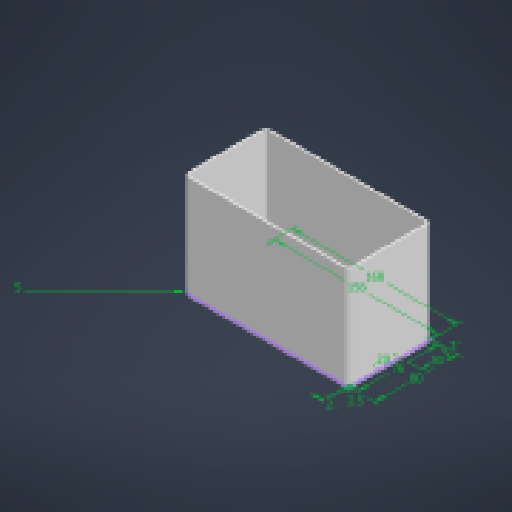
# Autodesk Inventor part: Base
Saved by Autodesk Inventor 2026.1 (Build 301233020, 233B)
## iProperties
Created: 2025-10-20
Part Number: Base
Material: Generic
Document SubType Name: Modeling
Designer: Nathan
Density: 1 g/cm^3
Appearance: Default
Author: Nathan
Autodesk Inventor part; units mm, degrees
ref_plane "YZ Plane" through (0, 0, 0) normal (1, 0, 0) x (0, 1, 0)
ref_plane "XZ Plane" through (0, 0, 0) normal (0, 1, 0) x (-1, 0, 0)
ref_plane "XY Plane" through (0, 0, 0) normal (0, 0, 1) x (1, 0, 0)
sketch "BaseBottom" plane through (0, 0, 0) normal (0, 1, 0) x (-1, 0, 0)
  line L0 (108.8151, 0.0203) -> (-41.1849, 0.0203)
  line L1 (-46.1849, -4.9797) -> (-46.1849, -74.9797)
  line L2 (-41.1849, -79.9797) -> (108.8151, -79.9797)
  line L3 (113.8151, -74.9797) -> (113.8151, -4.9797)
  arc A0 (113.8151, -4.9797) -> (108.8151, 0.0203) centre (108.8151, -4.9797) ccw
  arc A1 (108.8151, -79.9797) -> (113.8151, -74.9797) centre (108.8151, -74.9797) ccw
  arc A2 (-46.1849, -74.9797) -> (-41.1849, -79.9797) centre (-41.1849, -74.9797) ccw
  arc A3 (-41.1849, 0.0203) -> (-46.1849, -4.9797) centre (-41.1849, -4.9797) ccw
  line L4 (109.3151, -1.9797) -> (-41.6849, -1.9797)
  line L5 (-44.1849, -4.4797) -> (-44.1849, -75.4797)
  line L6 (-41.6849, -77.9797) -> (109.3151, -77.9797)
  line L7 (111.8151, -75.4797) -> (111.8151, -4.4797)
  arc A4 (-41.6849, -1.9797) -> (-44.1849, -4.4797) centre (-41.6849, -4.4797) ccw
  arc A5 (-44.1849, -75.4797) -> (-41.6849, -77.9797) centre (-41.6849, -75.4797) ccw
  arc A6 (109.3151, -77.9797) -> (111.8151, -75.4797) centre (109.3151, -75.4797) ccw
  arc A7 (111.8151, -4.4797) -> (109.3151, -1.9797) centre (109.3151, -4.4797) ccw
  line L8 (-46.1849, -29.9797) -> (-44.1849, -29.9797)
  line L9 (-44.1849, -29.9797) -> (-44.1849, -49.9797)
  line L10 (-44.1849, -49.9797) -> (-46.1849, -49.9797)
  line L11 (-46.1849, -49.9797) -> (-46.1849, -29.9797)
  point P0 (-46.1849, -79.9797)
  point P1 (-46.1849, 0.0203)
  point P2 (113.8151, -79.9797)
  point P3 (-44.1849, -77.9797)
  point P4 (-44.1849, -1.9797)
  point P5 (111.8151, -77.9797)
  point P6 (-45.1849, -49.9797)
  dimension "d2" = 160
  dimension "d3" = 80
  dimension "d4" = 5
  dimension "d6" = 156
  dimension "d7" = 76
  dimension "d8" = 2
  dimension "d9" = 2
  dimension "d10" = 2.5
  dimension "d11" = 20
  dimension "d12" = 30
  constraints: 24 end point, 16 point on circle, 16 tangent, 14 point on line, 8 centre point, 6 equal radius, 6 parallel, 3 horizontal, 3 perpendicular, 1 midpoint
  measures "d2" distance of point (113.815, -79.98) point (-46.185, -79.98)
  measures "d3" distance of point (-46.185, -79.98) point (-46.185, 0.02)
  measures "d4" radius of A0
  measures "d6" distance of point (111.815, -77.98) point (-44.185, -77.98)
  measures "d7" distance of point (-44.185, -77.98) point (-44.185, -1.98)
  measures "d8" distance between parallel lines of L2 L6
  measures "d9" distance between parallel lines of L1 L5
  measures "d10" radius of A4
  measures "d11" distance of L8.end L9.end
  measures "d12" distance from line of L2 point (-45.185, -49.98)
extrude "BaseFloor" add sketch "BaseBottom" against normal blind 2
extrude "BaseFill" add sketch "BaseBottom" along normal blind 98
extrude "BaseHollow" cut sketch "BaseBottom" along normal blind 100 contours L5 A4 L4 A7 L7 A6 L6 A5
